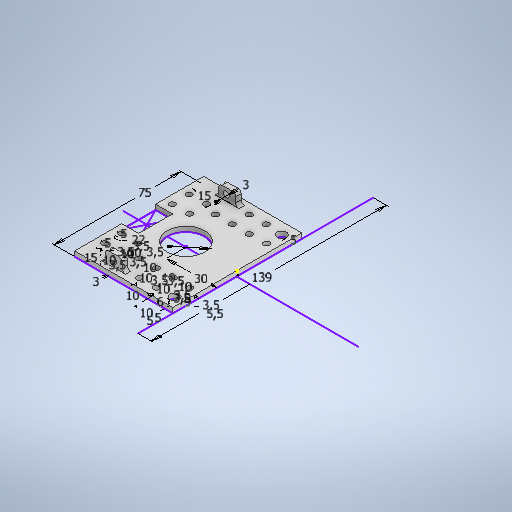
# Autodesk Inventor part: étage_BAU
Saved by Autodesk Inventor 2025.1 (Build 291241000, 241)
## iProperties
Created: 2024-09-16
Part Number: étage_BAU
Material: Générique
Document SubType Name: Modeling
Designer: chass
Density: 1 g/cm^3
Appearance: Par défaut
Author: chass
## iProperties of the stored document toit_Impression 3D.ipt
Created: 2024-09-16
Part Number: toit_Impression 3D
Material: Générique
Document SubType Name: Modeling
Designer: chass
Density: 1 g/cm^3
Appearance: Par défaut
Author: chass
Autodesk Inventor part; units mm, degrees
ref_plane "YZ Plane" through (0, 0, 0) normal (1, 0, 0) x (0, 1, 0)
ref_plane "XZ Plane" through (0, 0, 0) normal (0, 1, 0) x (-1, 0, 0)
ref_plane "XY Plane" through (0, 0, 0) normal (0, 0, 1) x (1, 0, 0)
sketch "Esquisse1" plane through (0, 0, 0) normal (0, 1, 0) x (-1, 0, 0)
  line L0 (57.9966, -37.2402) -> (57.9966, 37.7598)
  circle A0 centre (52.9966, 25.0001) radius 1.75
  circle A1 centre (52.9966, 15.0001) radius 1.75
  line L1 (67, 0.0502) -> (-72, 0.0502)
  circle A2 centre (43, 25.2598) radius 1.75
  circle A3 centre (43, 15.2598) radius 1.75
  circle A4 centre (52.9966, -24.8996) radius 1.75
  circle A5 centre (52.9966, -14.8996) radius 1.75
  circle A6 centre (43, -25.1593) radius 1.75
  circle A7 centre (43, -15.1593) radius 1.75
  line L2 (0, 58.3407) -> (0, -80.6593)
  circle A8 centre (5, 31.7598) radius 2.75
  circle A9 centre (5, 22.7598) radius 1.75
  circle A10 centre (15, 32.5) radius 1.75
  circle A11 centre (15, 22.5) radius 1.75
  circle A12 centre (25, 32.5) radius 1.75
  circle A13 centre (25, 22.5) radius 1.75
  circle A14 centre (35, 22.5) radius 1.75
  circle A15 centre (5, -31.6593) radius 2.75
  circle A16 centre (5, -22.6593) radius 1.75
  circle A17 centre (15, -32.3995) radius 1.75
  circle A18 centre (15, -22.3995) radius 1.75
  circle A19 centre (25, -32.3995) radius 1.75
  circle A20 centre (25, -22.3995) radius 1.75
  circle A21 centre (35, -22.3995) radius 1.75
  line L3 (58, 10) -> (48, 10)
  line L4 (48, 10) -> (48, -10)
  line L5 (48, -10) -> (58, -10)
  line L6 (58, -10) -> (58, 10)
  line L7 (58, 10) -> (48, -10)
  line L8 (48, 10) -> (58, -10)
  line L9 (57.9966, 37.7598) -> (0, 37.7598)
  line L10 (0, -38.4609) -> (57.9966, -38.4609)
  line L11 (57.9966, -38.4609) -> (57.9966, 37.7598)
  line L12 (57.9966, 37.7598) -> (0, 37.7598)
  line L13 (0, 37.7598) -> (0, -38.4609)
  circle A22 centre (30, 0.0502) radius 11
  line L14 (42.9966, -35.3694) -> (42.9966, -32.3694)
  line L15 (42.9966, -32.3694) -> (33, -32.3694)
  line L16 (42.9966, -32.3694) -> (33, -35.5523)
  line L17 (42.9966, -35.3694) -> (33, -32.3694)
  line L18 (33, -32.3694) -> (33, -35.5523)
  line L19 (33, -35.5523) -> (42.9966, -35.3694)
  line L20 (42.9966, 31.7598) -> (42.9966, 34.7598)
  line L21 (42.9966, 34.7598) -> (32.9966, 34.7598)
  line L22 (42.9966, 34.7598) -> (32.9966, 31.7598)
  line L23 (42.9966, 31.7598) -> (32.9966, 34.7598)
  line L24 (32.9966, 34.7598) -> (32.9966, 31.7598)
  line L25 (32.9966, 31.7598) -> (42.9966, 31.7598)
  point P0 (0, 0)
  point P1 (0, 0)
  point P2 (0, 0)
  point P3 (53, 0)
  point P4 (57.9966, -10)
  point P5 (57.9966, 10)
  point P6 (38.783, -33.8694)
  point P7 (42.5405, 34.5217)
  point P8 (42.9966, -33.8694)
  point P9 (42.9966, 33.2598)
  point P10 (37.9983, -35.4609)
  dimension "d3" = 3.5
  dimension "d4" = 3.5
  dimension "d7" = 10
  dimension "d9" = 3.5
  dimension "d10" = 3.5
  dimension "d12" = 10
  dimension "d13" = 10
  dimension "d16" = 5
  dimension "d17" = 5
  dimension "d19" = 5.5
  dimension "d20" = 3.5
  dimension "d21" = 3.5
  dimension "d22" = 3.5
  dimension "d23" = 3.5
  dimension "d24" = 3.5
  dimension "d26" = 3.5
  dimension "d27" = 5
  dimension "d28" = 5
  dimension "d31" = 10
  dimension "d32" = 10
  dimension "d33" = 10
  dimension "d35" = 10
  dimension "d36" = 10
  dimension "d38" = 10
  dimension "d40" = 10
  dimension "d70" = 9
  dimension "d72" = 5
  dimension "d73" = 6
  dimension "d77" = 22
  dimension "d80" = 139
  dimension "d81" = 75
  dimension "d83" = 15
  dimension "d85" = 3
  dimension "d86" = 15
  dimension "d87" = 3
  dimension "d115" = 30
  constraints: 48 end point, 23 centre point, 11 symmetric about line, 3 midpoint, 3 point on line, 2 parallel, 1 coincident, 1 horizontal, 1 perpendicular, 1 vertical, 17 other
  measures "d3" diameter of A0
  measures "d4" diameter of A1
  measures "d7" distance of A0.centre A1.centre
  measures "d9" diameter of A2
  measures "d10" diameter of A3
  measures "d12" distance of A0.centre A2.centre
  measures "d13" distance of A3.centre A1.centre
  measures "d16" distance from line of L0 A1.centre
  measures "d17" distance from line of L0 A0.centre
  measures "d19" diameter of A8
  measures "d20" diameter of A9
  measures "d21" diameter of A10
  measures "d22" diameter of A11
  measures "d23" diameter of A12
  measures "d24" diameter of A13
  measures "d26" diameter of A14
  measures "d27" distance from line of L2 A8.centre
  measures "d28" distance from line of L2 A9.centre
  measures "d31" horizontal distance of A8.centre A10.centre
  measures "d32" horizontal distance of A9.centre A11.centre
  measures "d33" distance of A11.centre A10.centre
  measures "d35" distance of A10.centre A12.centre
  measures "d36" distance of A11.centre A13.centre
  measures "d38" distance of A13.centre A12.centre
  measures "d40" distance of A14.centre A13.centre
  measures "d70" distance of A9.centre A8.centre
  measures "d72" distance from line of L13 A15.centre
  measures "d73" distance from line of L9 A8.centre
  measures "d77" diameter of A22
  measures "d80" distance of L2.start L2.end
  measures "d81" distance of L0.start L0.end
  measures "d83" distance from line of L0 point (42.997, -33.869)
  measures "d85" distance between parallel lines of L9 L21
  measures "d86" distance from line of L0 L21.start
  measures "d87" distance from line of L10 point (37.998, -35.461)
  measures "d115" distance from line of L2 A22.centre
extrude "Extrusion1" add sketch "Esquisse1" along normal blind 3 contours L8 L7 L1 L0 | L5 L7 L8 | L1 L7 L0 | L4 L1 L8 L7 | L8 L1 L7 | L7 L1 L8 L3 | L4 L8 L1
sketch "Esquisse4" plane through (0, 3, 0) normal (0, 1, 0) x (1, 0, 0)
  point P0 (0, 0)
sketch "Esquisse5" plane through (0, 0, 0) normal (0, -1, 0) x (1, 0, 0)
  point P0 (0, 0)
sketch "Esquisse6" plane through (0, 0, 0) normal (0, -1, 0) x (1, 0, 0)
  point P0 (0, 0)
sketch "Esquisse7" plane through (0, 0, 0) normal (0, -1, 0) x (1, 0, 0)
  point P0 (0, 0)
sketch "Esquisse8" plane through (0, 0, 0) normal (0, -1, 0) x (1, 0, 0)
  point P0 (0, 0)
extrude "Extrusion5" cut sketch "Esquisse1" along normal blind 3 contours L8 L7 L1 L0 | L5 L7 L8 | L1 L7 L0 | L4 L1 L8 L7 | L8 L1 L7 | L7 L1 L8 L3 | L4 L8 L1 | A22 L1 | L1 A22
extrude "Extrusion7" add sketch "Esquisse1" along normal blind 3 contours L11 L10 L2 L1 A22 L4 L5 L0 | L3 L4 L1 A22 L2 L9 L0 | L17 L16 L14 | L19 L16 L17 | L16 L17 L15 | L16 L18 L17 | L23 L22 L20 | L25 L22 L23 | L22 L23 L21 | L22 L24 L23
extrude "Extrusion8" add sketch "Esquisse1" along normal blind 10 contours L23 L22 L20 | L25 L22 L23 | L22 L23 L21 | L22 L24 L23
extrude "Extrusion9" add sketch "Esquisse1" along normal blind 10 contours L17 L16 L14 | L19 L16 L17 | L16 L17 L15 | L16 L18 L17
sketch "Esquisse10" plane through (-42.9966, 3, -35.3694) normal (-0.0183, 0, -0.9998) x (-0.9998, 0, 0.0183)
  line L0 (1.2831, 0) -> (1.2831, 7) projected
  line L1 (1.2831, 7) -> (-10, 0)
  line L2 (-43.046, 0) -> (14.9409, 0) projected
  line L3 (-9.9983, 7) -> (0, 7) projected
  line L4 (1.2831, 0) -> (-9.9983, 7)
  circle A0 centre (-4.3576, 3.5) radius 1.75
  point P0 (-42.3423, -3)
  dimension "d108" = 3.5
  constraints: 4 end point, 2 point on line, 1 centre point, 1 coincident, 1 midpoint
  measures "d108" diameter of A0
sketch "Esquisse11" plane through (-42.9966, 3, 34.7598) normal (0, 0, 1) x (1, 0, 0)
  line L0 (10, 0) -> (10, 7) projected
  line L1 (10, 7) -> (-0.0034, 0)
  line L2 (-1.7534, 0) -> (1.7466, 0) projected
  line L3 (42.9966, 0) -> (-15, 0) projected
  line L4 (0, 0) -> (0, 7) projected
  line L5 (10, 0) -> (0, 7)
  circle A0 centre (4.9992, 3.5006) radius 1.75
  point P0 (42.9966, -3)
  dimension "d109" = 3.5
  constraints: 4 end point, 2 point on line, 1 centre point, 1 coincident, 1 midpoint
  measures "d109" diameter of A0
extrude "Extrusion10" cut sketch "Esquisse11" against normal blind 3.5 contours A0 L1 L5 | L5 L1 A0 | L1 L5 A0 | L1 A0 L5
extrude "Extrusion11" cut sketch "Esquisse10" against normal blind 3.5 contours A0 L1 L4 | L4 L1 A0 | L1 L4 A0 | A0 L4 L1
fillet "Congé10" radius 2 8 edges at (-42.9966, 10, -33.8694) (-42.9966, 3, -33.8694) (-33, 10, -33.9609) (-33, 3, -33.9609) (-32.9966, 10, 33.2598) (-32.9966, 3, 33.2598) (-42.9966, 10, 33.2598) (-42.9966, 3, 33.2598)
